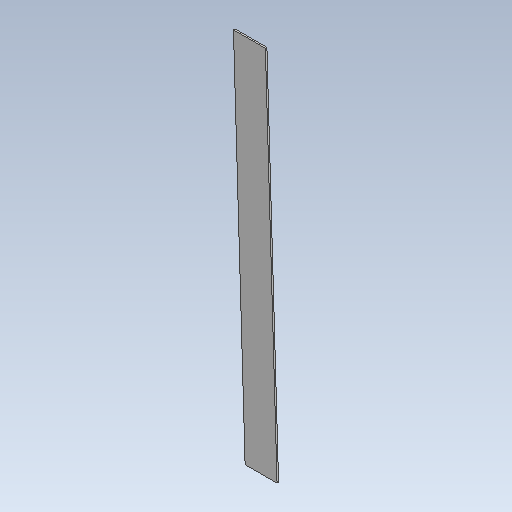
# Autodesk Inventor part: bottom_side_plate
Saved by Autodesk Inventor 2020.3 (Build 243373010, 373A)
## iProperties
Created: 2021-01-30
Part Number: bottom_side_plate
Material: Generic
Document SubType Name: Modeling
Designer: kardo
Density: 1 g/cm^3
Appearance: Default
Mass: 9.39146 g
Surface Area: 164.485 cm^2
Volume: 9.39146 cm^3
Author: kardo
Autodesk Inventor part; units mm, degrees
ref_plane "YZ Plane" through (0, 0, 0) normal (1, 0, 0) x (0, 1, 0)
ref_plane "XZ Plane" through (0, 0, 0) normal (0, 1, 0) x (-1, 0, 0)
ref_plane "XY Plane" through (0, 0, 0) normal (0, 0, 1) x (1, 0, 0)
derived "base_sketch.ipt"
sketch "stringer" plane through (0, 0, 0) normal (1, 0, 0) x (0, 1, 0)
  line L0 (-306, 11.475) -> (0, 0)
  line L1 (-306, 31.875) -> (-306, 11.475)
  line L2 (-412.4622, 0) -> (310.4457, 0)
  line L3 (0, -13.6228) -> (0, 64.3297)
  line L4 (0, 0) -> (122.4, 8.559)
  line L5 (-306, 31.875) -> (-153, 45.9) construction
  line L6 (-153, 45.9) -> (0, 45.9) construction
  line L7 (0, 45.9) -> (102, 45.9) construction
  line L8 (102, 45.9) -> (204, 35.7) construction
  line L9 (122.4, 8.559) -> (204, 14.2651) construction
  spline S0 degree 4 poles (-306, 31.875) (-229.6805, 38.871) (-153.0004, 41.6957) (-76.5755, 45.9) (0, 45.9) knots 0 0 0 0 0 1 1 1 1 1
  spline S1 degree 4 poles (0, 45.9) (51.0599, 45.9) (102.0004, 42.8427) (153.143, 40.7857) (204, 35.7) knots 0 0 0 0 0 1 1 1 1 1
  spline S2 degree 4 poles (122.4, 8.559) (129.6243, 9.0642) (155.3021, 10.8598) (183.5774, 20.1745) (192.0601, 27.4338) (204, 35.7) knots 0 0 0 0 0 0.281346 1 1 1 1 1
  point P0 (-153, 41.6925)
  point P1 (102, 42.84)
  point P2 (163.2, 15.056)
  point P3 (187.68, 24.9131)
sketch "stringer_inside" plane through (0, 0, 0) normal (1, 0, 0) x (0, 1, 0)
  line L0 (-306, 31.875) -> (-306, 11.475)
  line L1 (0, 0) -> (122.4, 8.559)
  line L2 (-306, 14.025) -> (-193.8, 14.025)
  line L3 (112.2, 23.3566) -> (112.2, 33.6972)
  line L4 (0, 45.9) -> (56.7636, 45.9) construction
  line L5 (56.7636, 45.9) -> (112.2, 33.6972) construction
  line L6 (112.2, 42.3143) -> (112.2, 7.8458) construction
  line L7 (0, -13.6228) -> (0, 64.3297)
  line L8 (-193.8, 14.025) -> (112.2, 23.3566)
  line L9 (-193.8, 14.025) -> (0, 13.529)
  line L10 (17.2125, 13.5685) -> (112.2, 16.4652)
  line L11 (0, 13.529) -> (-0.1952, 19.9291) construction
  line L12 (17.2125, 13.5685) -> (17.0025, 20.4535) construction
  spline S0 degree 4 poles (0, 45.9) (51.0599, 45.9) (102.0004, 42.8427) (153.143, 40.7857) (204, 35.7) knots 0 0 0 0 0 1 1 1 1 1
  spline S1 degree 3 poles (0, 45.9) (37.8279, 45.9) (75.6167, 40.2679) (112.2, 33.6972) knots 0 0 0 0 1 1 1 1
  spline S2 degree 4 poles (0, 13.529) (2.1516, 13.5235) (6.4547, 13.5125) (10.7595, 13.3717) (15.0615, 13.5029) (17.2125, 13.5685) knots 0 0 0 0 0 0.5 1 1 1 1 1
  point P0 (56.7636, 42.2391)
sketch "bulkhead_main" plane through (0, 0, 0) normal (0, 1, 0) x (-1, 0, 0)
  line L0 (0, 19.935) -> (28.764, 19.935)
  line L1 (28.764, 19.935) -> (28.764, 13.529)
  line L2 (28.764, 13.529) -> (62.322, 13.529)
  line L3 (0, 0) -> (-11.5056, 0)
  line L4 (-11.5056, 0) -> (-11.5056, -2.4868)
  line L5 (-11.5056, -2.4868) -> (-34.5168, -2.4868)
  line L6 (-34.5168, -2.4868) -> (-57.528, 27.54)
  line L7 (19.176, 46.818) -> (62.322, 46.818)
  line L8 (0, 19.935) -> (0, 0)
  line L9 (86.7165, 0) -> (-84.045, 0)
  line L10 (0, -13.6228) -> (0, 64.3297)
  line L11 (62.322, 46.818) -> (62.322, 13.529)
  line L12 (0, 35.7) -> (-57.528, 27.54) construction
  line L13 (-11.5056, -2.4868) -> (0, -2.4868) construction
  line L14 (0, -2.4868) -> (0, 0) construction
  spline S0 degree 4 poles (-57.528, 27.54) (-46.0483, 34.2051) (-30.6129, 40.5281) (-11.2214, 45.0414) (8.3201, 46.818) (15.5662, 46.818) (19.176, 46.818) knots 0 0 0 0 0 0.630279 0.815816 1 1 1 1 1
  point P0 (0, 45.9)
  point P1 (-38.352, 36.72)
  point P2 (-19.176, 42.5952)
  point P3 (0, 13.529)
sketch "bulkhead_F1" plane through (0, 56.1, 0) normal (0, 1, 0) x (-1, 0, 0)
  line L0 (19.176, 46.818) -> (62.322, 46.818)
  line L1 (-34.5168, -2.4868) -> (-57.528, 27.54)
  line L2 (-11.5056, -2.4868) -> (-34.5168, -2.4868)
  line L3 (-11.5056, 0) -> (-11.5056, -2.4868)
  line L4 (0, 0) -> (-11.5056, 0)
  line L5 (62.322, 46.818) -> (62.322, 13.529)
  line L6 (28.764, 19.935) -> (28.764, 13.529)
  line L7 (-37.5231, 1.4361) -> (-11.5056, 1.4361)
  line L8 (-11.5056, 1.4361) -> (-11.5056, 3.9229)
  line L9 (-11.5056, 3.9229) -> (0, 3.9229)
  line L10 (0, 3.9229) -> (0, 21.6458)
  line L11 (0, 21.6458) -> (28.764, 21.6458)
  line L12 (28.764, 21.6458) -> (28.764, 14.7544)
  line L13 (28.764, 14.7544) -> (62.322, 14.7544)
  line L14 (62.322, 43.2359) -> (19.176, 43.2359)
  line L15 (-57.528, 27.54) -> (-37.5231, 1.4361)
  line L16 (0, 45.9) -> (0, 44.8052) construction
  line L17 (-19.176, 42.5952) -> (-19.176, 41.8654) construction
  line L18 (-38.352, 36.72) -> (-38.352, 36.3551) construction
  line L19 (0, 19.935) -> (0, 0)
  line L20 (0, 44.8052) -> (0, 42.3179)
  line L21 (0, 35.7) -> (-57.528, 27.54) construction
  line L22 (-11.5056, 1.4361) -> (0, 1.4361) construction
  line L23 (0, 1.4361) -> (0, 3.9229) construction
  spline S0 degree 4 poles (-57.528, 27.54) (-46.0483, 34.2051) (-30.6129, 40.5281) (-11.2214, 45.0414) (8.3201, 46.818) (15.5662, 46.818) (19.176, 46.818) knots 0 0 0 0 0 0.630279 0.815816 1 1 1 1 1
  spline S1 degree 3 poles (-57.528, 27.54) (-39.1506, 37.8756) (-19.5945, 42.9173) (0, 44.8052) knots 0 0 0 0 1 1 1 1
  spline S2 degree 2 poles (0, 42.3179) (9.5715, 43.2359) (19.176, 43.2359) knots 0 0 0 1 1 1
  point P0 (0, 14.7544)
sketch "bulkhead_front" plane through (0, 112.2, 33.6972) normal (0, 1, 0) x (-1, 0, 0)
  line L0 (-40.5295, -28.3381) -> (-11.5056, -28.3381)
  line L1 (-11.5056, -28.3381) -> (-11.5056, -25.8514)
  line L2 (-11.5056, -25.8514) -> (0, -25.8514)
  line L3 (19.176, 13.1208) -> (62.322, 13.1208)
  line L4 (-11.5056, -36.1839) -> (-34.5168, -36.1839)
  line L5 (-11.5056, -33.6972) -> (-11.5056, -36.1839)
  line L6 (0, -33.6972) -> (-11.5056, -33.6972)
  line L7 (-34.5168, -36.1839) -> (-57.528, -6.1572)
  line L8 (0, -13.7621) -> (28.764, -13.7621)
  line L9 (28.764, -20.1682) -> (62.322, -20.1682)
  line L10 (28.764, -13.7621) -> (28.764, -20.1682)
  line L11 (62.322, 13.1208) -> (62.322, -20.1682)
  line L12 (0, -13.7621) -> (0, -33.6972)
  line L13 (0, -25.8514) -> (0, -10.3406)
  line L14 (0, -10.3406) -> (62.322, -10.3406)
  line L15 (19.176, 0.918) -> (62.322, 0.918)
  line L16 (-38.352, 1.8276) -> (-38.352, 3.0228) construction
  line L17 (-19.176, 6.5076) -> (-19.176, 8.898) construction
  line L18 (0, 8.6171) -> (0, 12.2028) construction
  line L19 (-40.5295, -28.3381) -> (-57.528, -6.1572)
  line L20 (0, 8.6171) -> (0, 0)
  line L21 (0, 2.0028) -> (-57.528, -6.1572) construction
  line L22 (-11.5056, -28.3381) -> (0, -28.3381) construction
  line L23 (0, -28.3381) -> (0, -25.8514) construction
  spline S0 degree 4 poles (-57.528, -6.1572) (-46.0483, 0.508) (-30.6129, 6.8309) (-11.2214, 11.3442) (8.3201, 13.1208) (15.5662, 13.1208) (19.176, 13.1208) knots 0 0 0 0 0 0.630279 0.815816 1 1 1 1 1
  spline S1 degree 3 poles (-57.528, -6.1572) (-39.0789, 3.4175) (-19.5173, 7.5799) (0, 8.6171) knots 0 0 0 0 1 1 1 1
  spline S2 degree 3 poles (0, 0) (6.37, 0.918) (12.773, 0.918) (19.176, 0.918) knots 0 0 0 0 1 1 1 1
sketch "bulkhead_F2" plane through (0, 158.1, 33.6972) normal (0, 1, 0) x (-1, 0, 0)
  line L0 (19.176, 13.1208) -> (62.322, 13.1208)
  line L1 (62.322, 13.1208) -> (62.322, -20.1682)
  line L2 (0, -33.6972) -> (-11.5056, -33.6972)
  line L3 (-11.5056, -36.1839) -> (-34.5168, -36.1839)
  line L4 (-11.5056, -33.6972) -> (-11.5056, -36.1839)
  line L5 (-34.5168, -36.1839) -> (-57.528, -6.1572)
  line L6 (0, 5.8272) -> (0, -20.0113)
  line L7 (0, -20.0113) -> (-11.5056, -20.0113)
  line L8 (-11.5056, -20.0113) -> (-11.5056, -21.8764)
  line L9 (-11.5056, -21.8764) -> (-35.9142, -21.8764)
  line L10 (-35.9142, -21.8764) -> (-48.8988, -4.9332)
  line L11 (-57.528, -8.9984) -> (-57.528, -6.1572) construction
  line L12 (-38.352, 3.0228) -> (-38.352, -0.9966) construction
  line L13 (-19.176, 8.898) -> (-19.176, 3.7072) construction
  line L14 (0, 12.2028) -> (0, 5.8272) construction
  line L15 (0, 2.0028) -> (-57.528, -6.1572) construction
  line L16 (0, 19.4965) -> (0, 13.1208) construction
  line L17 (0, 13.1208) -> (-57.528, 13.1208) construction
  line L18 (-57.528, 13.1208) -> (-57.528, 15.9621) construction
  line L19 (-57.528, 15.9621) -> (0, 19.4965) construction
  line L20 (-38.352, 17.1402) -> (-38.352, 13.1208) construction
  line L21 (-19.176, 18.3184) -> (-19.176, 13.1208) construction
  line L22 (-48.8988, -4.9332) -> (-48.8988, -1.5617) construction
  line L23 (-48.8988, 16.4923) -> (-48.8988, 13.1208) construction
  line L24 (-11.5056, -21.8764) -> (0, -21.8764) construction
  line L25 (0, -21.8764) -> (0, -20.0113) construction
  spline S0 degree 4 poles (-57.528, -6.1572) (-46.0483, 0.508) (-30.6129, 6.8309) (-11.2214, 11.3442) (8.3201, 13.1208) (15.5662, 13.1208) (19.176, 13.1208) knots 0 0 0 0 0 0.630279 0.815816 1 1 1 1 1
  spline S1 degree 3 poles (-57.528, -8.9984) (-39.0792, 0.5819) (-19.5206, 4.7923) (0, 5.8272) knots 0 0 0 0 1 1 1 1
sketch "bulkhead_B1" plane through (0, -102, 0) normal (0, 1, 0) x (-1, 0, 0)
  line L0 (19.176, 46.818) -> (62.322, 46.818)
  line L1 (0, 19.935) -> (0, 0)
  line L2 (62.322, 46.818) -> (62.322, 13.529)
  line L3 (0, 5.6919) -> (-27.3644, 38.3035)
  line L4 (62.322, 44.7066) -> (19.176, 44.7066)
  line L5 (-38.352, 36.72) -> (-38.352, 34.6086) construction
  line L6 (-19.176, 42.5952) -> (-19.176, 40.4838) construction
  line L7 (0, 45.9) -> (0, 43.7886) construction
  line L8 (19.176, 46.818) -> (19.176, 44.7066) construction
  line L9 (0, 19.935) -> (28.764, 19.935)
  line L10 (28.764, 19.935) -> (28.764, 13.529)
  line L11 (28.764, 13.529) -> (62.322, 13.529)
  line L12 (62.322, 13.7901) -> (28.764, 13.7901)
  line L13 (28.764, 13.7901) -> (28.764, 16.8245)
  line L14 (28.764, 16.8245) -> (0, 16.8245)
  line L15 (0, 16.8245) -> (0, 5.6919)
  spline S0 degree 4 poles (-57.528, 27.54) (-46.0483, 34.2051) (-30.6129, 40.5281) (-11.2214, 45.0414) (8.3201, 46.818) (15.5662, 46.818) (19.176, 46.818) knots 0 0 0 0 0 0.630279 0.815816 1 1 1 1 1
  spline S1 degree 3 poles (19.176, 44.7066) (-0.1981, 44.9447) (-19.6083, 41.6917) (-38.352, 34.6086) knots 0 0 0 0 1 1 1 1
  point P0 (0, 3.825)
  point P1 (0, 13.7901)
sketch "bulkhead_B2" plane through (0, -204, 0) normal (0, 1, 0) x (-1, 0, 0)
  line L0 (19.176, 46.818) -> (62.322, 46.818)
  line L1 (0, 19.935) -> (28.764, 19.935)
  line L2 (28.764, 13.529) -> (62.322, 13.529)
  line L3 (28.764, 19.935) -> (28.764, 13.529)
  line L4 (62.322, 46.818) -> (62.322, 13.529)
  line L5 (0, 9.5169) -> (0, 14.025)
  line L6 (0, 14.025) -> (62.322, 14.025)
  line L7 (0, 9.5169) -> (-21.5668, 35.2191)
  line L8 (62.322, 40.0294) -> (19.176, 40.0294)
  line L9 (-19.176, 35.8066) -> (-19.176, 42.5952) construction
  line L10 (-38.352, 36.72) -> (-38.352, 29.9314) construction
  line L11 (19.176, 46.818) -> (19.176, 40.0294) construction
  line L12 (0, 45.9) -> (0, 39.1114) construction
  spline S0 degree 4 poles (-57.528, 27.54) (-46.0483, 34.2051) (-30.6129, 40.5281) (-11.2214, 45.0414) (8.3201, 46.818) (15.5662, 46.818) (19.176, 46.818) knots 0 0 0 0 0 0.630279 0.815816 1 1 1 1 1
  spline S1 degree 3 poles (19.176, 40.0294) (-0.1981, 40.2675) (-19.6083, 37.0145) (-38.352, 29.9314) knots 0 0 0 0 1 1 1 1
  point P0 (0, 0)
  point P1 (0, 7.65)
sketch "transom" plane through (0, -306, 31.875) normal (0, 1, 0) x (-1, 0, 0)
  line L0 (19.176, 14.943) -> (62.322, 14.943)
  line L1 (62.322, 14.943) -> (62.322, -18.346)
  line L2 (28.764, -18.346) -> (62.322, -18.346)
  line L3 (0, -18.5331) -> (-13.7701, -2.1226)
  line L4 (0, -18.5331) -> (0, -17.85)
  line L5 (0, -17.85) -> (62.322, -17.85)
  line L6 (62.322, 0.918) -> (19.176, 0.918)
  line L7 (19.176, 14.943) -> (19.176, 0.918) construction
  line L8 (-19.176, -3.3048) -> (-19.176, 10.7202) construction
  line L9 (-38.352, 4.845) -> (-38.352, -9.18) construction
  line L10 (0, 14.025) -> (0, 0) construction
  line L11 (0, 0) -> (0, -20.4)
  spline S0 degree 4 poles (-57.528, -4.335) (-46.0483, 2.3301) (-30.6129, 8.6531) (-11.2214, 13.1664) (8.3201, 14.943) (15.5662, 14.943) (19.176, 14.943) knots 0 0 0 0 0 0.630279 0.815816 1 1 1 1 1
  spline S1 degree 3 poles (19.176, 0.918) (-0.1981, 1.1561) (-19.6083, -2.0969) (-38.352, -9.18) knots 0 0 0 0 1 1 1 1
  point P0 (0, -31.875)
sketch "stinger_bottom_liner" plane through (0, 0, 0) normal (1, 0, 0) x (0, 1, 0)
  line L0 (0, -2.4868) -> (56.1, 1.4361)
  line L1 (56.1, 1.4361) -> (112.2, 5.359)
  line L2 (112.2, 5.359) -> (122.4, 6.0723)
  line L3 (0, -2.4868) -> (0, 0) construction
  line L4 (56.1, 1.4361) -> (56.1, 3.9229) construction
  line L5 (112.2, 5.359) -> (112.2, 7.8458) construction
  line L6 (158.1, 11.8207) -> (158.1, 13.6858) construction
  line L7 (0, 0) -> (122.4, 8.559)
  spline S0 degree 4 poles (122.4, 6.0723) (129.6678, 6.5805) (155.5572, 8.3909) (183.6316, 19.8242) (192.0814, 26.863) (204, 35.7) knots 0 0 0 0 0 0.280728 1 1 1 1 1
  spline S1 degree 4 poles (122.4, 8.559) (129.6243, 9.0642) (155.3021, 10.8598) (183.5774, 20.1745) (192.0601, 27.4338) (204, 35.7) knots 0 0 0 0 0 0.281346 1 1 1 1 1
  point P0 (163.2, 13.3976)
  point P1 (187.68, 24.2914)
  point P2 (187.68, 24.9131)
  point P3 (163.2, 15.056)
ref_plane "Work Plane1" through (0, -193.8, 14.025) normal (0, -0.0304813, 0.9995353) x (0, 0.9995353, 0.0304813)
sketch "Sketch11" plane through (0, -193.8, 14.025) normal (0, -0.0304813, 0.9995353) x (0, 0.9995353, 0.0304813)
  line L0 (0, 0) -> (306.1423, 0) construction
  line L1 (193.8901, 0) -> (193.8901, 28.764) construction
  line L2 (0, 27.564) -> (306.1423, 27.564)
  line L3 (306.1423, 27.564) -> (306.1423, 2)
  line L4 (306.1423, 2) -> (0, 2)
  line L5 (0, 2) -> (0, 27.564)
  point P0 (193.2824, 0)
  dimension "d1" = 2
  dimension "d4" = 1.2
  constraints: 8 end point, 3 parallel, 2 point on line, 1 perpendicular
  measures "d1" distance between parallel lines of L0 L4
  measures "d4" distance from line of L1.end L2
extrude "Extrusion1" add sketch "Sketch11" along normal blind 1.2
equation "\"d1\" = stringer_thickness"
equation "\"d4\" = decking_thickness"
equation "\"d5\" = decking_thickness"
equation "\"stringer_thickness\" = 2"
equation "\"decking_thickness\" = 1.2"
body "Solid1"
